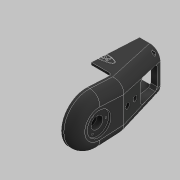
# Autodesk Inventor part: Część12
Saved by Autodesk Inventor 2021 (Build 250183000, 183)
## iProperties
Created: 2021-09-29
Part Number: Część12
Material: Kauczuk
Document SubType Name: Modeling
Designer: marci
Density: 0.93 g/cm^3
Appearance: Kauczuk — czarny
Author: marci
Autodesk Inventor part; units mm, degrees
ref_plane "YZ Plane" through (0, 0, 0) normal (1, 0, 0) x (0, 1, 0)
ref_plane "XZ Plane" through (0, 0, 0) normal (0, 1, 0) x (-1, 0, 0)
ref_plane "XY Plane" through (0, 0, 0) normal (0, 0, 1) x (1, 0, 0)
sketch "Szkic1" plane through (0, 0, 0) normal (1, 0, 0) x (0, 1, 0)
  line L0 (10, -182.6) -> (70, -182.6)
  line L1 (40, -182.6) -> (0, -182.6)
  line L2 (0, -182.6) -> (80, -182.6)
  arc A0 (87.4333, -42.517) -> (-7.4333, -42.517) centre (40, -40) ccw
  line L3 (0, -182.6) -> (-7.4333, -42.517)
  line L4 (80, -182.6) -> (87.4333, -42.517)
  point P0 (0, 0)
  point P1 (0, -40)
  point P2 (0, -89.6806)
  point P3 (80, -40)
  point P4 (80, 0)
  point P5 (40, 0)
  point P6 (69.8888, -177.435)
  point P7 (80, -177.435)
  point P8 (80, -40)
  point P9 (0, -40)
  point P10 (10.1112, -177.435)
  dimension "d14" = 60
  dimension "d16" = 182.6
  dimension "d21" = 80
  dimension "d22" = 95
  dimension "d23" = 142.6
  dimension "d24" = 40
  constraints: 10 end point, 3 horizontal, 2 point on circle, 2 tangent, 1 centre point, 1 midpoint
  measures "d14" distance of L0.start L0.end
  measures "d16" distance from line of point (0, 0) L0
  measures "d21" distance of L1.end L2.end
  measures "d22" diameter of A0
  measures "d23" distance from line of L0 A0.centre
  measures "d24" horizontal distance of point (0, 0) A0.centre
extrude "Wyciągnięcie proste1" add sketch "Szkic1" along normal blind 130
ref_plane "Płaszczyzna konstrukcyjna1" through (130, 40, 7.5) normal (0, -1, 0) x (1, 0, 0)
sketch "Szkic2" plane through (130, 40, 7.5) normal (0, -1, 0) x (1, 0, 0)
  line L0 (-65, -190.1) -> (-65, 20.9163) construction
  line L1 (-65, -190.1) -> (-25, -190.1)
  line L2 (-130, -190.1) -> (0, -190.1) projected
  line L3 (0, -50.017) -> (0, 0) projected
  line L4 (0, 0) -> (0, -95)
  line L5 (0, -95) -> (-25, -190.1)
  line L6 (-65, -190.1) -> (-105, -190.1)
  line L7 (-130, 0) -> (-130, -95)
  line L8 (-130, -95) -> (-105, -190.1)
  line L9 (0, 0) -> (-130, 0)
  line L10 (0, -190.1) -> (0, -50.017) projected
  line L11 (0, -95) -> (0, -190.1)
  line L12 (0, -190.1) -> (-130, -190.1)
  line L13 (-130, -190.1) -> (-130, -95)
  point P0 (-130, -7.5)
  point P1 (0, 27)
  dimension "d27" = 40
  dimension "d28" = 95
  constraints: 22 end point, 3 perpendicular, 3 symmetric about line, 2 point on line, 2 vertical
  measures "d27" distance of L0.start L1.end
  measures "d28" distance of L3.end L4.end
extrude "Wyciągnięcie proste2" cut sketch "Szkic2" along normal mid plane 130 contours L5 L10 L2 | L2 L13 L8
fillet "Zaokrąglenie1" radius 20 10 edges at (130, -6.2398, -65.0085) (130, 86.2398, -65.0085) (130, 40, 7.5) (117.5, 82.5232, -135.05) (117.5, -2.5232, -135.05) (12.5, 82.5232, -135.05) (12.5, -2.5232, -135.05) (0, -6.2398, -65.0085) (0, 86.2398, -65.0085) (0, 40, 7.5)
sketch "Szkic3" plane through (84.5991, 80, -182.6) normal (0, 0, -1) x (-1, 0, 0)
  point P0 (84.5991, -80)
sketch "Szkic4" plane through (84.5991, 80, -182.6) normal (0, 0, -1) x (-1, 0, 0)
  line L0 (47.5991, -12) -> (-8.4009, -12)
  line L1 (-8.4009, -12) -> (-8.4009, -68)
  line L2 (-8.4009, -68) -> (47.5991, -68)
  line L3 (47.5991, -68) -> (47.5991, -12)
  line L4 (47.5991, -12) -> (-8.4009, -68) construction
  line L5 (-8.4009, -12) -> (47.5991, -68) construction
  line L6 (-20.4009, -19.7583) -> (-20.4009, -60.2417) projected
  line L7 (39.1981, 0) -> (0, 0) projected
  point P0 (84.5991, -80)
  point P1 (19.5991, -40)
  dimension "d37" = 56
  dimension "d38" = 56
  dimension "d39" = 40
  dimension "d40" = 40
  constraints: 12 end point, 2 midpoint, 2 parallel, 1 horizontal, 1 perpendicular
  measures "d37" distance of L2.end L1.end
  measures "d38" distance of L1.end L0.end
  measures "d39" distance from line of point (19.599, -40) L6
  measures "d40" distance from line of L7 point (19.599, -40)
ref_plane "Płaszczyzna konstrukcyjna2" through (65, 0, 0) normal (-1, 0, 0) x (0, 0, 1)
sketch "Szkic5" plane through (65, 0, 0) normal (-1, 0, 0) x (0, 0, 1)
  arc A0 (-42.517, -7.4333) -> (-42.517, 87.4333) centre (-40, 40) ccw projected
  circle A1 centre (-40, 40) radius 40
  point P0 (0, 0)
  dimension "d41" = 80
  constraints: 1 centre point, 1 coincident
  measures "d41" diameter of A1
extrude "Wyciągnięcie proste3" cut sketch "Szkic5" along normal mid plane 86
sketch "Szkic6" plane through (65, 0, 0) normal (-1, 0, 0) x (0, 0, 1)
  arc A0 (-42.517, -7.4333) -> (-42.517, 87.4333) centre (-40, 40) ccw projected
  circle A1 centre (-40, 40) radius 47.5
  point P0 (0, 0)
  point P1 (-42.517, 87.4333)
  constraints: 1 centre point, 1 coincident
extrude "Wyciągnięcie proste4" cut sketch "Szkic6" against normal mid plane 80
extrude "Wyciągnięcie proste5" cut sketch "Szkic4" against normal through all
ref_plane "Płaszczyzna konstrukcyjna3" through (37, 40, -182.6) normal (0, 1, 0) x (1, 0, 0)
sketch "Szkic7" plane through (37, 40, -182.6) normal (0, 1, 0) x (1, 0, 0)
  line L0 (71, -182.6) -> (71, -102.6) projected
  line L1 (71, -182.6) -> (71, -92.6)
  line L2 (56, -95.1) -> (56, -104.2301) projected
  line L3 (71, -182.6) -> (161, -182.6) construction
  line L4 (71, -92.6) -> (-15, -92.6)
  line L5 (-15, -92.6) -> (-15, -182.6)
  line L6 (71, -142.6) -> (-15, -142.6)
  line L7 (-15, -102.6) -> (-15, -182.6) projected
  point P0 (-37, -182.6)
  point P1 (68, -182.6)
  point P2 (-15, -142.6)
  dimension "d49" = 90
  dimension "d50" = 90
  dimension "d51" = 90
  dimension "d52" = 90
  dimension "d53" = 86
  dimension "d54" = 40
  constraints: 10 end point, 3 perpendicular, 1 horizontal, 1 midpoint, 1 parallel, 1 point on line
  measures "d49" distance of L0.start L1.end
  measures "d50" angle of L3 L1
  measures "d51" distance of L4.end L5.end
  measures "d52" angle of L5 L4
  measures "d53" distance of L1.end L4.end
  measures "d54" distance from line of L0.start L6
extrude "Wyciągnięcie proste6" cut sketch "Szkic7" along normal mid plane 80
sketch "Szkic8" plane through (22, 0, -90) normal (0, 0, 1) x (1, 0, 0)
  line L0 (86, 80) -> (0, 80) projected
  line L1 (0, 0) -> (86, 0) projected
  line L2 (86, 80) -> (0, 80)
  line L3 (0, 80) -> (0, 0)
  line L4 (0, 0) -> (86, 0)
  line L5 (86, 0) -> (86, 80)
  point P0 (-22, 0)
  constraints: 8 end point, 2 parallel, 1 horizontal, 1 perpendicular
loft "Wyciągnięcie złożone1" cut profiles "Szkic8", "Szkic4"
sketch "Szkic10" plane through (37, 80, -182.6) normal (0, -1, 0) x (1, 0, 0)
  line L0 (71, 92.6) -> (-15, 92.6) projected
  line L1 (-12, 140.083) -> (68, 140.083) projected
  line L2 (-12, 140.083) -> (-12, 92.6)
  line L3 (68, 116.9826) -> (68, 142.6) projected
  line L4 (68, 140.083) -> (68, 116.9826)
  line L5 (-12, 140.083) -> (68, 140.083)
  line L6 (68, 140.083) -> (68, 92.6)
  line L7 (-12, 92.6) -> (68, 92.6)
  line L8 (-12, 140.083) -> (68, 140.083) projected
  point P0 (-37, 182.6)
  constraints: 10 end point, 3 perpendicular, 2 point on line, 1 parallel, 1 vertical
extrude "Wyciągnięcie proste7" cut sketch "Szkic10" against normal through all both and the other way through all
sketch "Szkic11" plane through (45.4009, 80, -182.6) normal (0, 0.9985951, -0.0529887) x (1, 0, 0)
  point P0 (-45.4009, -178.1044)
ref_plane "Płaszczyzna konstrukcyjna5" through (52.5, 84.9137, -90) normal (0, -1, 0) x (1, 0, 0)
sketch "Szkic14" plane through (52.5, 84.9137, -90) normal (0, -1, 0) x (1, 0, 0)
  line L0 (22.795, 14.5574) -> (22.795, 12.2635)
  line L1 (22.795, 12.2635) -> (21.3835, 12.2635)
  ellipse E0 centre (30.5552, 14.4374) end of major axis (30.5552, 16.9591) minor radius 1.8166 (31.7717, 12.5647) -> (32.0564, 13.0174) ccw
  line L2 (30.2552, 14.1374) -> (30.2552, 12.3968)
  ellipse E1 centre (30.5552, 14.4374) end of major axis (30.5552, 16.478) minor radius 1.3356 (29.504, 13.1787) -> (31.5945, 13.1559) ccw
  arc A0 (32.4717, 12.8457) -> (28.588, 12.8733) centre (30.5001, 8.6651) ccw
  ellipse E2 centre (30.5552, 14.4374) end of major axis (30.5552, 16.9591) minor radius 1.8166 (29.0382, 13.05) -> (29.3386, 12.5647) ccw
  line L3 (30.8552, 14.1374) -> (30.8552, 12.3968)
  arc A1 (27.3206, 15.4265) -> (23.1913, 16.325) centre (21.11, -3.1784) ccw
  arc A2 (27.882, 16.068) -> (27.3206, 15.4265) centre (30.8788, 12.8795) ccw
  line L4 (28.2291, 15.765) -> (23.577, 15.765) construction
  arc A3 (27.882, 16.068) -> (23.1913, 16.325) centre (25.0093, 6.5676) ccw
  arc A4 (18.7347, 7.3964) -> (19.2526, 10.0425) centre (16.5271, 9.2022) ccw
  ellipse E3 centre (30.5552, 14.4374) end of major axis (30.5552, 16.9591) minor radius 1.8166 (29.3386, 16.3102) -> (28.8973, 13.4065) ccw
  line L5 (30.2552, 14.7374) -> (27.5257, 14.7374)
  line L6 (30.2552, 14.1374) -> (27.5257, 14.1374)
  line L7 (30.2552, 14.7374) -> (30.2552, 16.478)
  arc A5 (30.2552, 13.6656) -> (28.2291, 13.1099) centre (30.4328, 9.0468) ccw
  line L8 (30.8552, 14.7374) -> (30.8552, 16.478)
  ellipse E4 centre (30.5552, 14.4374) end of major axis (30.5552, 16.478) minor radius 1.3356 (31.6256, 15.6577) -> (29.3552, 13.5416) ccw
  ellipse E5 centre (30.5552, 14.4374) end of major axis (27.4924, 14.4374) minor radius 2.0406
  arc A6 (28.4821, 15.9396) -> (32.5968, 15.9586) centre (30.5163, 20.9559) ccw
  arc A7 (28.2291, 15.765) -> (32.8812, 15.765) centre (30.5552, 20.6528) ccw
  line L9 (28.2291, 15.765) -> (32.8812, 15.765) construction
  line L10 (19.093, 8.4256) -> (19.0757, 6.1218)
  line L11 (19.093, 8.4256) -> (20.3419, 8.4256)
  line L12 (19.0757, 6.1218) -> (21.3621, 6.1047)
  arc A8 (21.3621, 6.1047) -> (23.1913, 9.4412) centre (20.3201, 8.8456) ccw
  arc A9 (20.3419, 8.4256) -> (20.3419, 9.4412) centre (20.089, 8.9334) ccw
  arc A10 (23.1913, 9.4412) -> (21.5414, 11.5115) centre (20.3201, 8.8456) ccw
  arc A11 (21.3835, 12.2635) -> (21.5414, 11.5115) centre (21.4935, 11.894) ccw
  arc A12 (20.3201, 14.4752) -> (20.3419, 9.4412) centre (21.3706, 11.9627) ccw
  line L13 (20.3201, 14.4752) -> (20.5414, 14.5567)
  line L14 (20.5414, 14.5567) -> (22.795, 14.5574)
  circle A13 centre (-25.0705, 12.499) radius 1.0042
  arc A14 (-25.9395, 11.1945) -> (-25.8255, 6.2929) centre (-24.3438, 8.7795) ccw
  arc A15 (-26.5669, 12.0324) -> (-26.3588, 5.3939) centre (-24.3438, 8.7795) ccw
  arc A16 (-26.5669, 12.0324) -> (-25.9395, 11.1945) centre (-25.0705, 12.499) ccw
  ellipse E6 centre (30.5552, 14.4374) end of major axis (30.5552, 16.9591) minor radius 1.8166 (32.0997, 15.765) -> (31.7717, 16.3102) ccw
  ellipse E7 centre (30.5552, 14.4374) end of major axis (30.5552, 16.478) minor radius 1.3356 (31.7352, 13.4817) -> (31.7426, 15.3715) ccw
  ellipse E8 centre (30.5552, 14.4374) end of major axis (30.5552, 16.9591) minor radius 1.8166 (32.1851, 13.324) -> (32.2037, 15.4968) ccw
  arc A17 (32.7752, 13.0315) -> (30.8552, 13.6497) centre (30.4328, 9.0468) ccw
  line L15 (30.8552, 14.1374) -> (33.5847, 14.1374)
  line L16 (30.8552, 14.7374) -> (33.5847, 14.7374)
  line L17 (30.8552, 14.7374) -> (33.5847, 14.7374)
  line L18 (34.0461, 14.7374) -> (34.0711, 14.7374)
  line L19 (34.0461, 14.7374) -> (34.0711, 14.7374)
  line L20 (42.5187, 2.1682) -> (42.5187, 23.4584)
  line L21 (71.9675, 8.4128) -> (71.9843, 6.1658)
  arc A18 (64.6955, 9.4412) -> (64.6955, 8.4256) centre (64.9484, 8.9334) ccw
  arc A19 (63.496, 11.5115) -> (61.8461, 9.4412) centre (64.7173, 8.8456) ccw
  arc A20 (61.8461, 9.4412) -> (63.6753, 6.1047) centre (64.7173, 8.8456) ccw
  line L22 (79.4135, 15.0446) -> (75.744, 18.3181)
  line L23 (76.315, 2.138) -> (76.2088, 2.1633)
  line L24 (54.7822, 14.7374) -> (54.7822, 16.478)
  line L25 (72.6827, 4.5451) -> (72.8428, 4.507)
  ellipse E9 centre (54.4822, 14.4374) end of major axis (54.4822, 16.478) minor radius 1.3356 (55.6822, 13.5416) -> (53.4118, 15.6577) ccw
  ellipse E10 centre (54.4822, 14.4374) end of major axis (57.545, 14.4374) minor radius 2.0406
  arc A21 (68.0271, 7.7472) -> (72.6827, 4.5451) centre (74.8004, 12.6095) ccw
  arc A22 (66.3027, 7.3964) -> (72.4555, 3.3075) centre (75.7129, 14.8828) ccw
  line L26 (54.1822, 14.7374) -> (54.1822, 16.478)
  circle A23 centre (74.5065, 3.3075) radius 1.5974
  circle A24 centre (74.5065, 3.3075) radius 2.0511
  line L27 (62.2424, 14.5574) -> (62.2424, 12.2635)
  line L28 (48.4119, 19.6561) -> (48.4119, 2.1682) construction
  line L29 (83.2687, 7.0657) -> (99.9206, 7.0659)
  line L30 (85.3525, 6.2671) -> (85.3525, 14.5148)
  line L31 (65.9617, 6.1218) -> (63.6753, 6.1047)
  line L32 (65.9444, 8.4256) -> (65.9617, 6.1218)
  arc A25 (109.1037, 13.703) -> (108.5497, 12.6716) centre (110.1079, 12.499) ccw
  line L33 (108.4183, 12.7197) -> (108.5497, 12.6716)
  line L34 (62.2424, 12.2635) -> (63.6539, 12.2635)
  arc A26 (82.4144, 15.5369) -> (79.4135, 15.0446) centre (84.95, -9.3126) ccw
  line L35 (95.9893, 19.6561) -> (48.4119, 19.6561) construction
  line L36 (48.4119, 2.1682) -> (95.9893, 2.1682) construction
  arc A27 (76.315, 2.138) -> (100.4281, 1.5548) centre (89.9711, 67.9731) ccw
  arc A28 (76.5576, 3.3075) -> (100.2424, 2.7346) centre (89.9711, 67.9731) ccw
  line L37 (73.9024, 8.4401) -> (73.9194, 6.1813)
  line L38 (73.9024, 8.4401) -> (75.2144, 8.4399)
  line L39 (75.3081, 6.1917) -> (73.9194, 6.1813)
  line L40 (75.3105, 14.5565) -> (73.9035, 14.5569)
  arc A29 (75.2144, 8.4399) -> (75.2151, 12.3966) centre (74.6541, 10.4183) ccw
  arc A30 (75.3081, 6.1917) -> (75.3105, 14.5565) centre (74.7636, 10.3742) ccw
  line L41 (83.2687, 6.2515) -> (83.2687, 7.0657)
  arc A31 (99.9204, 13.0203) -> (99.9206, 7.0659) centre (99.9205, 10.0431) ccw
  arc A32 (109.1037, 13.703) -> (86.9846, 18.0089) centre (86.4822, -43.5357) ccw
  line L42 (101.1285, 13.0199) -> (102.5137, 13.0199)
  line L43 (85.3525, 14.5148) -> (98.6063, 13.0199)
  arc A33 (100.6331, 10.7271) -> (100.524, 10.825) centre (99.9205, 10.0431) ccw
  line L44 (99.9205, 11.0308) -> (100.524, 11.0308)
  line L45 (100.524, 9.0554) -> (99.9205, 9.0554)
  line L46 (100.524, 11.0308) -> (100.524, 9.0554)
  line L47 (101.1285, 13.0199) -> (99.9204, 13.0203)
  line L48 (101.1285, 13.0199) -> (99.9204, 13.0203)
  line L49 (102.5137, 13.0199) -> (98.6063, 13.0199)
  line L50 (102.5135, 8.5803) -> (102.5135, 8.4482)
  circle A34 centre (110.1079, 12.499) radius 1.0042
  arc A35 (110.9769, 11.1945) -> (111.6043, 12.0324) centre (110.1079, 12.499) ccw
  arc A36 (99.9205, 11.0308) -> (99.9205, 9.0554) centre (99.9205, 10.0431) ccw
  circle A37 centre (101.557, 2.3767) radius 0.8592
  arc A38 (108.4183, 12.7197) -> (87.163, 15.8489) centre (90.4839, -35.3472) ccw
  arc A39 (110.8629, 6.2929) -> (110.9769, 11.1945) centre (109.3812, 8.7795) ccw
  arc A40 (111.3962, 5.3939) -> (111.6043, 12.0324) centre (109.3812, 8.7795) ccw
  line L51 (85.3525, 6.2671) -> (93.6002, 6.2671) construction
  arc A41 (102.6003, 3.2269) -> (110.8629, 6.2929) centre (98.404, 27.2015) ccw
  arc A42 (102.9058, 2.2194) -> (111.3962, 5.3939) centre (98.404, 27.2015) ccw
  line L52 (95.9893, 2.1682) -> (95.9893, 19.6561) construction
  line L53 (85.3525, 6.2671) -> (83.2687, 6.2515)
  line L54 (102.6003, 3.2269) -> (102.608, 3.2366)
  arc A43 (102.9058, 2.2194) -> (102.608, 3.2366) centre (101.557, 2.3767) ccw
  arc A44 (100.2474, 2.7354) -> (100.4711, 1.5616) centre (101.557, 2.3767) ccw
  arc A45 (87.163, 15.8489) -> (86.9846, 18.0089) centre (85.5591, 16.8038) ccw
  line L55 (68.1241, 12.3603) -> (68.1248, 14.5567)
  arc A46 (69.2252, 11.5104) -> (69.2252, 6.1451) centre (70.6841, 8.8277) ccw
  arc A47 (70.3924, 9.4405) -> (70.394, 14.556) centre (69.5053, 11.9985) ccw
  line L56 (70.4228, 8.4133) -> (71.9675, 8.4128)
  line L57 (71.9843, 6.1658) -> (69.2252, 6.1451)
  line L58 (100.2424, 2.7346) -> (100.2474, 2.7353)
  line L59 (100.4281, 1.5548) -> (100.4711, 1.5616)
  arc A48 (70.3924, 9.4405) -> (70.4228, 8.4133) centre (70.8165, 8.939) ccw
  arc A49 (90.5858, 18.0091) -> (75.744, 18.3181) centre (82.5232, -12.6616) ccw
  ellipse E11 centre (54.4822, 14.4374) end of major axis (54.4822, 16.9591) minor radius 1.8166 (52.981, 13.0174) -> (53.2657, 12.5647) ccw
  ellipse E12 centre (54.4822, 14.4374) end of major axis (54.4822, 16.9591) minor radius 1.8166 (55.6988, 12.5647) -> (55.9992, 13.05) ccw
  line L60 (54.7822, 14.1374) -> (54.7822, 12.3968)
  line L61 (54.1822, 14.1374) -> (54.1822, 12.3968)
  ellipse E13 centre (54.4822, 14.4374) end of major axis (54.4822, 16.478) minor radius 1.3356 (53.4429, 13.1559) -> (55.5334, 13.1787) ccw
  arc A50 (56.4494, 12.8733) -> (52.5657, 12.8457) centre (54.5373, 8.6651) ccw
  line L62 (73.9031, 12.3968) -> (73.9035, 14.5569)
  circle A51 centre (85.5591, 16.8038) radius 1.3392
  line L63 (73.9031, 12.3968) -> (75.2151, 12.3966)
  arc A52 (61.8461, 16.325) -> (57.7168, 15.4265) centre (63.9274, -3.1784) ccw
  arc A53 (57.7168, 15.4265) -> (57.1554, 16.068) centre (54.1586, 12.8795) ccw
  arc A54 (61.8461, 16.325) -> (57.1554, 16.068) centre (60.0281, 6.5676) ccw
  line L64 (56.8083, 15.765) -> (61.4604, 15.765) construction
  arc A55 (69.1321, 11.1912) -> (68.0271, 7.7472) centre (70.5757, 8.8287) ccw
  arc A56 (68.2218, 12.6004) -> (65.7848, 10.0425) centre (70.1099, 8.3618) ccw
  arc A57 (65.7848, 10.0425) -> (66.3027, 7.3964) centre (68.5103, 9.2022) ccw
  ellipse E14 centre (54.4822, 14.4374) end of major axis (54.4822, 16.9591) minor radius 1.8166 (56.1401, 13.4065) -> (55.6988, 16.3102) ccw
  line L65 (54.7822, 14.7374) -> (57.5117, 14.7374)
  line L66 (54.7822, 14.1374) -> (57.5117, 14.1374)
  arc A58 (56.8083, 13.1099) -> (54.7822, 13.6656) centre (54.6046, 9.0468) ccw
  arc A59 (54.1822, 13.6497) -> (52.2622, 13.0315) centre (54.6046, 9.0468) ccw
  ellipse E15 centre (54.4822, 14.4374) end of major axis (54.4822, 16.478) minor radius 1.3356 (53.2948, 15.3715) -> (53.3022, 13.4817) ccw
  ellipse E16 centre (54.4822, 14.4374) end of major axis (54.4822, 16.9591) minor radius 1.8166 (53.2657, 16.3102) -> (52.9377, 15.765) ccw
  ellipse E17 centre (54.4822, 14.4374) end of major axis (54.4822, 16.9591) minor radius 1.8166 (52.8337, 15.4968) -> (52.8523, 13.324) ccw
  arc A60 (63.496, 11.5115) -> (63.6539, 12.2635) centre (63.5439, 11.894) ccw
  arc A61 (64.6955, 9.4412) -> (64.7173, 14.4752) centre (63.6668, 11.9627) ccw
  line L67 (64.496, 14.5567) -> (62.2424, 14.5574)
  line L68 (64.7173, 14.4752) -> (64.496, 14.5567)
  arc A62 (52.1562, 15.765) -> (56.8083, 15.765) centre (54.4822, 20.6528) ccw
  line L69 (56.8083, 15.765) -> (52.1562, 15.765) construction
  arc A63 (52.4406, 15.9586) -> (56.5553, 15.9396) centre (54.5211, 20.9559) ccw
  line L70 (82.4144, 15.5369) -> (84.1882, 15.5369)
  arc A64 (84.1336, 18.0089) -> (84.1882, 15.5369) centre (85.5591, 16.8038) ccw
  line L71 (65.9444, 8.4256) -> (64.6955, 8.4256)
  line L72 (90.5858, 18.0091) -> (84.1336, 18.0089)
  line L73 (54.1822, 14.1374) -> (51.4527, 14.1374)
  line L74 (54.1822, 14.7374) -> (51.4527, 14.7374)
  line L75 (54.1822, 14.7374) -> (51.4527, 14.7374)
  line L76 (69.1321, 11.1912) -> (69.1503, 11.2022)
  line L77 (50.9913, 14.7374) -> (50.9663, 14.7374)
  line L78 (50.9913, 14.7374) -> (50.9663, 14.7374)
  line L79 (68.2218, 12.6004) -> (68.245, 12.6107)
  arc A65 (68.245, 12.6107) -> (69.1503, 11.2022) centre (69.931, 12.6991) ccw
  line L80 (68.1241, 12.3603) -> (69.2998, 12.3603)
  arc A66 (69.2252, 11.5104) -> (69.2998, 12.3603) centre (69.2998, 11.9321) ccw
  line L81 (70.394, 14.556) -> (68.1248, 14.5567)
  arc A67 (1.5725, -22.8881) -> (3.3687, -26.1646) centre (4.392, -23.473) ccw
  arc A68 (4.3706, -22.8881) -> (4.3706, -23.8855) centre (4.619, -23.3868) ccw
  arc A69 (3.1927, -20.8551) -> (1.5725, -22.8881) centre (4.392, -23.473) ccw
  line L82 (11.5135, -23.8969) -> (11.53, -26.1035)
  line L83 (-4.7308, -26.1868) -> (-4.5735, -26.2242)
  circle A70 centre (-2.9398, -27.4021) radius 1.5686
  circle A71 centre (-2.9398, -27.4021) radius 2.0141
  line L84 (-5.3642, -17.6873) -> (-5.3642, -15.978)
  arc A72 (-9.3026, -23.0423) -> (-4.7308, -26.1868) centre (-2.6512, -18.2675) ccw
  arc A73 (-10.9959, -23.3868) -> (-4.9539, -27.4021) centre (-1.7551, -16.0352) ccw
  arc A74 (-8.2174, -19.6604) -> (-9.3026, -23.0423) centre (-6.7999, -21.9803) ccw
  line L85 (-11.6199, -12.8571) -> (-11.6199, -30.0303) construction
  arc A75 (-11.5045, -20.7883) -> (-10.9959, -23.3868) centre (-8.8281, -21.6135) ccw
  line L86 (-1.1639, -28.5505) -> (-1.2682, -28.5257)
  line L87 (1.9617, -16.0319) -> (-1.2286, -13.7889)
  ellipse E18 centre (-5.6588, -17.9819) end of major axis (-2.6512, -17.9819) minor radius 2.0039
  ellipse E19 centre (-5.6588, -17.9819) end of major axis (-5.6588, -15.978) minor radius 1.3115 (-4.4804, -18.8615) -> (-6.71, -16.7836) ccw
  arc A76 (22.7166, -20.1167) -> (22.6095, -20.0205) centre (22.0168, -20.7883) ccw
  line L88 (24.6558, -26.0051) -> (24.6558, -17.9058)
  line L89 (24.6558, -26.0051) -> (22.6095, -26.0204)
  line L90 (22.6095, -23.7119) -> (22.0168, -23.7119)
  line L91 (22.6095, -26.0204) -> (22.6095, -23.7119)
  arc A77 (22.0168, -17.8647) -> (22.0168, -23.7119) centre (22.0168, -20.7883) ccw
  arc A78 (14.7945, -26.079) -> (14.7945, -17.8647) centre (14.2586, -21.9719) ccw
  arc A79 (14.7022, -23.8713) -> (14.7022, -19.9858) centre (14.1516, -21.9285) ccw
  line L92 (13.4138, -23.8713) -> (14.7022, -23.8713)
  line L93 (14.7945, -26.079) -> (13.4304, -26.0892)
  line L94 (13.4138, -23.8713) -> (13.4304, -26.0892)
  line L95 (1.9617, -17.8647) -> (1.9617, -20.1167)
  line L96 (1.9617, -20.1167) -> (3.3478, -20.1167)
  line L97 (5.614, -26.1478) -> (3.3687, -26.1646)
  line L98 (5.597, -23.8855) -> (5.614, -26.1478)
  arc A80 (6.5419, -15.3931) -> (1.9617, -16.0319) centre (7.5736, -39.529) ccw
  arc A81 (9.3754, -15.2556) -> (9.3139, -12.9655) centre (7.9141, -14.149) ccw
  line L99 (7.7393, -20.0205) -> (7.7393, -17.8647)
  line L100 (24.6585, -27.4719) -> (24.6555, -27.4719)
  arc A82 (24.9481, -28.4678) -> (24.6555, -27.4719) centre (23.6236, -28.3161) ccw
  circle A83 centre (23.6236, -28.3161) radius 0.8438
  line L101 (22.5152, -29.1233) -> (22.5574, -29.1166)
  arc A84 (22.3377, -27.9639) -> (22.5574, -29.1166) centre (23.6236, -28.3161) ccw
  line L102 (22.3328, -27.9647) -> (22.3377, -27.9639)
  arc A85 (31.0349, -17.194) -> (30.4908, -18.2068) centre (32.021, -18.3763) ccw
  line L103 (30.3618, -18.1596) -> (30.4908, -18.2068)
  line L104 (24.6558, -26.0051) -> (32.755, -26.0051) construction
  arc A86 (24.6585, -27.4719) -> (32.7592, -24.4684) centre (20.5391, -3.9361) ccw
  arc A87 (24.9481, -28.4678) -> (33.2866, -25.3544) centre (20.5391, -3.9361) ccw
  line L105 (35.1011, -30.0303) -> (35.1011, -12.8571) construction
  circle A88 centre (32.021, -18.3763) radius 0.9861
  arc A89 (32.7592, -24.4684) -> (32.8727, -19.6588) centre (31.3068, -22.028) ccw
  arc A90 (32.8727, -19.6588) -> (33.4915, -18.8324) centre (32.021, -18.3763) ccw
  arc A91 (33.2866, -25.3544) -> (33.4915, -18.8324) centre (31.3068, -22.028) ccw
  line L106 (22.6095, -19.8184) -> (22.6095, -21.7583)
  line L107 (24.6558, -17.9058) -> (24.6558, -17.8647)
  line L108 (24.5631, -17.8647) -> (24.6558, -17.8647)
  line L109 (14.7945, -17.8647) -> (13.4138, -17.8647)
  arc A92 (31.0349, -17.194) -> (9.3139, -12.9655) centre (8.8206, -73.4024) ccw
  line L110 (23.2028, -17.8647) -> (24.5631, -17.8647)
  line L111 (22.0168, -19.8184) -> (22.6095, -19.8184)
  line L112 (23.2028, -17.8647) -> (22.0168, -17.8647)
  line L113 (23.2028, -17.8647) -> (22.0168, -17.8647)
  line L114 (22.6095, -21.7583) -> (22.0168, -21.7583)
  arc A93 (22.0168, -19.8184) -> (22.0168, -21.7583) centre (22.0168, -20.7883) ccw
  arc A94 (30.3618, -18.1596) -> (9.3754, -15.2556) centre (13.108, -65.5636) ccw
  line L115 (24.5631, -22.2249) -> (24.5631, -22.3545)
  line L116 (13.4138, -19.9858) -> (14.7022, -19.9858)
  line L117 (6.5419, -15.3931) -> (6.5678, -15.3931)
  arc A95 (6.5142, -12.9655) -> (6.5678, -15.3931) centre (7.9141, -14.149) ccw
  line L118 (13.4138, -19.9858) -> (13.4138, -17.8647)
  ellipse E20 centre (-5.6588, -17.9819) end of major axis (-5.6588, -15.978) minor radius 1.3115 (-6.6795, -19.2404) -> (-4.6265, -19.2179) ccw
  arc A96 (-9.1114, -18.2765) -> (-11.5045, -20.7883) centre (-7.2573, -22.4388) ccw
  line L119 (-5.9534, -18.2765) -> (-5.9534, -19.9858)
  line L120 (-5.3642, -18.2765) -> (-5.3642, -19.9858)
  line L121 (-5.9534, -17.6873) -> (-5.9534, -15.978)
  arc A97 (8.8206, -20.8551) -> (8.8206, -26.1238) centre (10.2533, -23.4894) ccw
  line L122 (11.53, -26.1035) -> (8.8206, -26.1238)
  arc A98 (9.9665, -22.8881) -> (9.9665, -17.8647) centre (9.0946, -20.3764) ccw
  line L123 (9.9967, -23.8969) -> (11.5135, -23.8969)
  ellipse E21 centre (-5.6588, -17.9819) end of major axis (-5.6588, -15.5055) minor radius 1.7839 (-4.4642, -19.8209) -> (-4.1692, -19.3443) ccw
  arc A99 (9.9665, -22.8881) -> (9.9967, -23.8969) centre (10.3831, -23.3805) ccw
  arc A100 (6.4132, -12.9655) -> (-1.2286, -13.7889) centre (6.0469, -45.4396) ccw
  ellipse E22 centre (-5.6588, -17.9819) end of major axis (-5.6588, -15.5056) minor radius 1.7839 (-7.133, -19.3763) -> (-6.8535, -19.8209) ccw
  arc A101 (-2.4825, -17.0106) -> (-3.0338, -16.3806) centre (-5.9766, -19.5117) ccw
  arc A102 (1.5725, -16.1283) -> (-2.4825, -17.0106) centre (3.6163, -35.2806) ccw
  arc A103 (1.5725, -16.1283) -> (-3.0338, -16.3806) centre (-0.2127, -25.71) ccw
  circle A104 centre (7.9141, -14.149) radius 1.3151
  arc A105 (-3.7271, -19.5178) -> (-7.5409, -19.545) centre (-5.6047, -23.6503) ccw
  arc A106 (-9.0886, -18.2664) -> (-8.1996, -19.6496) centre (-7.433, -18.1795) ccw
  line L124 (-8.2174, -19.6604) -> (-8.1996, -19.6496)
  ellipse E23 centre (-5.6588, -17.9819) end of major axis (-5.6588, -15.5056) minor radius 1.7839 (-6.8535, -16.1428) -> (-7.1756, -16.6782) ccw
  ellipse E24 centre (-5.6588, -17.9819) end of major axis (-5.6588, -15.978) minor radius 1.3115 (-6.8249, -17.0645) -> (-6.8176, -18.9204) ccw
  line L125 (-5.9534, -17.6873) -> (-8.6338, -17.6873)
  line L126 (-5.9534, -17.6873) -> (-8.6338, -17.6873)
  line L127 (-5.9534, -18.2765) -> (-8.6338, -18.2765)
  arc A107 (-5.9534, -18.7554) -> (-7.8389, -19.3624) centre (-5.5387, -23.2754) ccw
  arc A108 (-7.6637, -16.4881) -> (-3.6231, -16.5068) centre (-5.6207, -11.5807) ccw
  arc A109 (-7.943, -16.6782) -> (-3.3746, -16.6782) centre (-5.6588, -11.8784) ccw
  ellipse E25 centre (-5.6588, -17.9819) end of major axis (-5.6588, -15.5055) minor radius 1.7839 (-4.0308, -18.9942) -> (-4.4642, -16.1428) ccw
  arc A110 (-3.3746, -19.2855) -> (-5.3642, -18.7398) centre (-5.5387, -23.2754) ccw
  line L128 (-5.3642, -18.2765) -> (-2.6838, -18.2765)
  arc A111 (3.1927, -20.8551) -> (3.3478, -20.1167) centre (3.2397, -20.4795) ccw
  line L129 (4.1747, -17.8647) -> (1.9617, -17.8647)
  line L130 (4.392, -17.9447) -> (4.1747, -17.8647)
  arc A112 (4.3706, -22.8881) -> (4.392, -17.9447) centre (3.3604, -20.412) ccw
  line L131 (-5.3642, -17.6873) -> (-2.6838, -17.6873)
  line L132 (-9.087, -17.6873) -> (-9.1114, -17.6873)
  line L133 (-9.087, -17.6873) -> (-9.1114, -17.6873)
  line L134 (-9.1114, -18.2765) -> (-9.0886, -18.2664)
  ellipse E26 centre (-5.6588, -17.9819) end of major axis (-5.6588, -15.5056) minor radius 1.7839 (-7.2777, -16.9415) -> (-7.2595, -19.0753) ccw
  line L135 (35.1011, -12.8571) -> (-11.6199, -12.8571) construction
  line L136 (-11.6199, -30.0303) -> (35.1011, -30.0303) construction
  arc A113 (-1.1639, -28.5505) -> (22.5152, -29.1233) centre (12.2464, 36.0996) ccw
  arc A114 (-0.9256, -27.4021) -> (22.3328, -27.9647) centre (12.2464, 36.0996) ccw
  line L137 (6.4132, -12.9655) -> (6.5142, -12.9655)
  line L138 (9.9665, -17.8647) -> (7.7393, -17.8647)
  line L139 (7.7393, -20.0205) -> (8.8938, -20.0205)
  arc A115 (8.8206, -20.8551) -> (8.8938, -20.0205) centre (8.8938, -20.441) ccw
  line L140 (5.597, -23.8855) -> (4.3706, -23.8855)
  point P0 (-52.5, 90)
  point P1 (-0.9256, -27.4021)
  point P2 (22.5152, -29.1233)
  point P3 (22.3377, -27.9639)
  point P4 (-11.5045, -20.7883)
  point P5 (-3.8876, -18.2765)
  point P6 (-5.9534, -19.9346)
  point P7 (-5.9534, -19.1247)
  point P8 (-5.3642, -19.1177)
  point P9 (-5.3642, -19.9346)
  point P10 (-4.3616, -18.2765)
  point P11 (-6.9561, -18.2765)
  point P12 (-7.4301, -18.2765)
  point P13 (-7.1699, -16.6656)
  point P14 (-7.4301, -17.6873)
  point P15 (-4.4928, -17.0645)
  point P16 (-5.3642, -17.1858)
  point P17 (-4.3616, -17.6873)
  point P18 (-5.9534, -17.1858)
  point P19 (-6.9561, -17.6873)
  point P20 (-5.9534, -16.886)
  point P21 (-5.9534, -16.0292)
  point P22 (-5.3642, -16.8902)
  point P23 (-4.6008, -16.7976)
  point P24 (-5.3642, -16.0292)
  point P25 (-4.1388, -16.6856)
  point P26 (-4.04, -16.9415)
  point P27 (-3.8876, -17.6873)
  dimension "d74" = 180
  constraints: 266 end point, 264 point on circle, 116 centre point, 80 symmetric about line, 10 point on line, 9 vertical, 3 coincident, 2 concentric, 2 perpendicular, 1 collinear, 170 other
  measures "d74" angle of L9 L4
extrude "Wyciągnięcie proste8" cut sketch "Szkic14" along normal blind 2 contours A69 A111 L96 L95 L129 L130 A112 A68 L140 L98 L97 A67 | L82 L122 A97 A115 L139 L99 L138 A98 A99 L123 | L83 A71 A73 A75 A96 L134 A106 L124 A74 A72 | A114 L102 A84 L101 A113 L86 A71 | A70 | L84 A109 E19 L131 | L84 E19 A108 | L121 L125 E24 A109 | E19 A110 L120 L128 | E25 A109 E18 L131 | A108 E19 L121 | L128 E18 A110 E25 | E25 E18 A108 | E26 L125 E18 A109 | A108 E18 E23 | L127 L119 A107 E24 | A105 E20 L120 | E26 A107 E18 L127 | E18 E21 A105 | L119 E20 A105 | E22 E18 A105 | L87 A100 L137 A95 L117 A80 | L89 L91 L90 A77 L112 L110 L108 L107 L88 | L93 L94 L92 A79 L116 L118 L109 A78 | A81 A92 A85 L103 A94 | A86 A89 A90 A91 A87 A82 L100 | A83 | A88 | A101 A103 A102 | A104
sketch "Szkic15" plane through (0, 0, 0) normal (-1, 0, 0) x (0, 0, 1)
  arc A0 (-41.4572, 12.5386) -> (-41.4572, 67.4614) centre (-40, 40) ccw projected
  circle A1 centre (-40, 40) radius 4
  circle A2 centre (-40, 40) radius 11.25
  point P0 (0, 0)
  dimension "d100" = 8
  dimension "d101" = 22.5
  constraints: 2 centre point, 2 coincident
  measures "d100" diameter of A1
  measures "d101" diameter of A2
extrude "Wyciągnięcie proste9" cut sketch "Szkic15" against normal blind 15 contours A1 | A2
sketch "Szkic16" plane through (15, 40, -40) normal (-1, 0, 0) x (0, 0, 1)
  circle A0 centre (0, 0) radius 11.25 projected
  circle A1 centre (0, 0) radius 4.15
  point P0 (40, -40)
  dimension "d104" = 8.3
  constraints: 1 centre point, 1 coincident
  measures "d104" diameter of A1
extrude "Wyciągnięcie proste10" cut sketch "Szkic16" against normal through all contours A1
sketch "Szkic17" plane through (0, 0, 0) normal (-1, 0, 0) x (0, 0, 1)
  circle A0 centre (-40, 40) radius 11.25 projected
  circle A1 centre (-40, 40) radius 22.5
  point P0 (0, 0)
  dimension "d107" = 45
  constraints: 1 centre point, 1 coincident
  measures "d107" diameter of A1
extrude "Wyciągnięcie proste11" cut sketch "Szkic17" against normal blind 4 contours A0 | A1
fillet "Zaokrąglenie2" radius 5 4 edges at (105, -2.4568, -90) (25, -2.4568, -90) (25, 82.4568, -90) (105, 82.4568, -90)
mirror "Odbij1" about plane through (65, 0, 0) normal (-1, 0, 0) of "Wyciągnięcie proste11", "Wyciągnięcie proste10", "Wyciągnięcie proste9"
sketch "Szkic19" plane through (130, 0, 0) normal (1, 0, 0) x (0, 0, -1)
  line L0 (182.6, 60.2417) -> (182.6, 19.7583) projected
  line L1 (135.6, 62) -> (169.6, 62)
  line L2 (174.6, 57) -> (174.6, 23)
  line L3 (169.6, 18) -> (135.6, 18)
  line L4 (130.6, 23) -> (130.6, 57)
  line L5 (130.6, 62) -> (174.6, 18) construction
  line L6 (174.6, 62) -> (130.6, 18) construction
  line L7 (130.6, 23) -> (135.6, 18)
  line L8 (130.6, 57) -> (135.6, 62)
  line L9 (169.6, 62) -> (174.6, 57)
  line L10 (169.6, 18) -> (174.6, 23)
  point P0 (0, 0)
  point P1 (152.6, 40)
  dimension "d114" = 44
  dimension "d115" = 44
  dimension "d116" = 5
  dimension "d117" = 5
  dimension "d118" = 5
  dimension "d119" = 5
  dimension "d120" = 5
  dimension "d121" = 5
  dimension "d122" = 5
  dimension "d123" = 5
  dimension "d124" = 8
  dimension "d125" = 1.7583
  constraints: 20 end point, 8 point on line, 2 midpoint, 2 parallel, 1 horizontal, 1 perpendicular
  measures "d114" distance of L5.end L6.end
  measures "d115" distance of L6.start L5.end
  measures "d116" distance of L4.start L6.end
  measures "d117" distance of L3.end L6.end
  measures "d118" distance of L4.end L5.start
  measures "d119" distance of L1.start L5.start
  measures "d120" distance of L1.end L6.start
  measures "d121" distance of L2.start L6.start
  measures "d122" distance of L3.start L5.end
  measures "d123" distance of L2.end L5.end
  measures "d124" distance between parallel lines of L0 L2
  measures "d125" distance from line of L0.end L3
extrude "Wyciągnięcie proste12" cut sketch "Szkic19" against normal blind 68.25
sketch "Szkic20" plane through (0, 0, 0) normal (-1, 0, 0) x (0, 0, 1)
  line L0 (-182.6, 19.7583) -> (-182.6, 60.2417) projected
  line L1 (-159.6, 18) -> (-145.6, 18)
  line L2 (-130.6, 33) -> (-130.6, 47)
  line L3 (-145.6, 62) -> (-159.6, 62)
  line L4 (-174.6, 47) -> (-174.6, 33)
  line L5 (-174.6, 18) -> (-130.6, 62) construction
  line L6 (-130.6, 18) -> (-174.6, 62) construction
  arc A0 (-145.6, 18) -> (-130.6, 33) centre (-145.6, 33) ccw
  arc A1 (-130.6, 47) -> (-145.6, 62) centre (-145.6, 47) ccw
  arc A2 (-159.6, 62) -> (-174.6, 47) centre (-159.6, 47) ccw
  arc A3 (-174.6, 33) -> (-159.6, 18) centre (-159.6, 33) ccw
  point P0 (0, 0)
  point P1 (-152.6, 40)
  dimension "d128" = 44
  dimension "d129" = 44
  dimension "d130" = 15
  dimension "d131" = 8
  constraints: 12 end point, 8 point on circle, 8 point on line, 8 tangent, 4 centre point, 3 equal radius, 2 midpoint, 2 parallel, 1 horizontal, 1 perpendicular
  measures "d128" distance of L6.end L5.end
  measures "d129" distance of L5.end L6.start
  measures "d130" radius of A0
  measures "d131" distance between parallel lines of L0 L4
extrude "Wyciągnięcie proste13" cut sketch "Szkic20" against normal blind 68.25
sketch "Szkic21" plane through (65, 0, 0) normal (-1, 0, 0) x (0, 0, 1)
  line L0 (-465.6875, -42.852) -> (373.4515, -42.852)
  line L1 (373.4515, -42.852) -> (373.4515, 144.5297)
  line L2 (373.4515, 144.5297) -> (-465.6875, 144.5297)
  line L3 (-465.6875, 144.5297) -> (-465.6875, -42.852)
  line L4 (-465.6875, -42.852) -> (373.4515, 144.5297) construction
  line L5 (373.4515, -42.852) -> (-465.6875, 144.5297) construction
  point P0 (0, 0)
  point P1 (-46.118, 50.8389)
  constraints: 12 end point, 2 midpoint, 2 parallel, 1 horizontal, 1 perpendicular
extrude "Wyciągnięcie proste14" cut sketch "Szkic21" along normal through all
sketch "Szkic22" plane through (126, 40, -40) normal (1, 0, 0) x (0, 0, -1)
  point P0 (-8.5, -14.7224)
  point P1 (-8.5, 14.7224)
  point P2 (17, 0)
hole "Otwór1" at (126, 25.2776, -31.5) at (126, 54.7224, -31.5) at (126, 40, -57) direction (-1, 0, 0) diameter 3.4 end through all
sketch "Szkic23" plane through (130, 14.9818, -87.5) normal (0.9671404, 0, -0.254243) x (-0.254243, 0, -0.9671404)
  circle A0 centre (10, 25.0182) radius 3
  circle A1 centre (30, 25.0182) radius 3
  line L0 (0, 0) -> (0, 50.0364) projected
  circle A2 centre (10, 25.0182) radius 5
  circle A3 centre (30, 25.0182) radius 5
  point P0 (-51.5732, -14.9818)
  dimension "d143" = 6
  dimension "d144" = 6
  dimension "d146" = 10
  dimension "d147" = 25.0182
  dimension "d148" = 20
  dimension "d149" = 25.0182
  dimension "d150" = 10
  dimension "d151" = 10
  constraints: 4 centre point, 2 coincident
  measures "d143" diameter of A0
  measures "d144" diameter of A1
  measures "d146" distance from line of L0 A0.centre
  measures "d147" vertical distance of L0.start A0.centre
  measures "d148" distance of A1.centre A0.centre
  measures "d149" vertical distance of L0.start A1.centre
  measures "d150" diameter of A2
  measures "d151" diameter of A3
extrude "Wyciągnięcie proste15" cut sketch "Szkic23" against normal through all contours A0 | A1
extrude "Wyciągnięcie proste16" cut sketch "Szkic23" against normal blind 8 contours A0 | A1 | A2 | A3
sketch "Szkic24" plane through (65, 0, 0) normal (-1, 0, 0) x (0, 0, 1)
  circle A0 centre (-174.6, 75) radius 1.65
  line L0 (-182.6, 68) -> (-182.6, 80) projected
  line L1 (-182.6, 60.2417) -> (-182.6, 19.7583) projected
  line L2 (-182.6, 40) -> (-157.2443, 40)
  circle A1 centre (-174.6, 5) radius 1.65
  point P0 (0, 0)
  dimension "d156" = 3.3
  dimension "d157" = 8
  dimension "d158" = 5
  constraints: 2 centre point, 2 end point, 1 horizontal, 1 midpoint, 1 symmetric about line, 1 other
  measures "d156" diameter of A0
  measures "d157" distance from line of L0 A0.centre
  measures "d158" vertical distance of L0.end A0.centre
extrude "Wyciągnięcie proste17" cut sketch "Szkic24" against normal through all
sketch "Szkic25" plane through (130, 0, 0) normal (1, 0, 0) x (0, 0, -1)
  circle A0 centre (174.6, 5) radius 1.65 projected
  line L0 (171.42, 5) -> (173.01, 7.754)
  line L1 (173.01, 7.754) -> (176.19, 7.754)
  line L2 (176.19, 7.754) -> (177.78, 5)
  line L3 (177.78, 5) -> (176.19, 2.246)
  line L4 (176.19, 2.246) -> (173.01, 2.246)
  line L5 (173.01, 2.246) -> (171.42, 5)
  circle A1 centre (174.6, 75) radius 1.65 projected
  line L6 (171.42, 75) -> (173.01, 77.754)
  line L7 (173.01, 77.754) -> (176.19, 77.754)
  line L8 (176.19, 77.754) -> (177.78, 75)
  line L9 (177.78, 75) -> (176.19, 72.246)
  line L10 (176.19, 72.246) -> (173.01, 72.246)
  line L11 (173.01, 72.246) -> (171.42, 75)
  point P0 (0, 0)
  dimension "d161" = 6.36
  dimension "d162" = 6.36
  constraints: 24 end point, 2 coincident, 26 other
  measures "d161" distance of L8.end L6.start
  measures "d162" distance of L2.end L0.start
extrude "Wyciągnięcie proste18" cut sketch "Szkic25" against normal blind 45 contours A0 | L0 L1 L2 L3 L4 L5 | A1 | L6 L7 L8 L9 L10 L11
equation "\"d117\" = d116"
equation "\"d118\" = d116"
equation "\"d119\" = d118"
equation "\"d120\" = d116"
equation "\"d121\" = d120"
equation "\"d122\" = d116"
equation "\"d123\" = d122"
